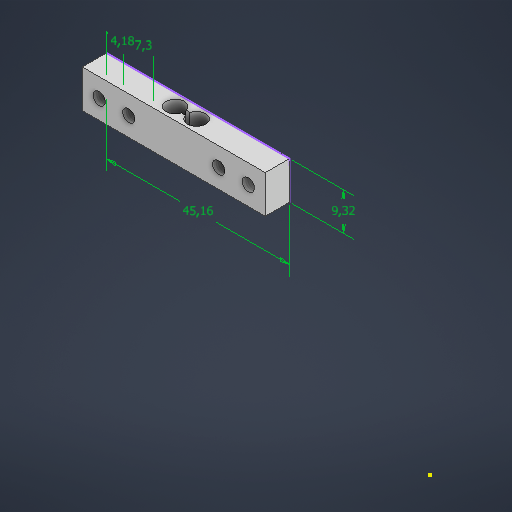
# Autodesk Inventor part: load_cell
Saved by Autodesk Inventor 2026 (Build 300175000, 175)
## iProperties
Created: 2025-04-15
Part Number: load_cell
Material: Generic
Document SubType Name: Modeling
Designer: Paul Juschitz
Density: 1 g/cm^3
Appearance: Default
load_cell_length: 45,160 mm
load_cell_width: 9,320 mm
load_cell_hole_inset: 4,180 mm
load_cell_hole_spacing: 7,300 mm
load_cell_height: 5,990 mm
Author: Paul Juschitz
Autodesk Inventor part; units mm, degrees
ref_plane "YZ Plane" through (0, 0, 0) normal (1, 0, 0) x (0, 1, 0)
ref_plane "XZ Plane" through (0, 0, 0) normal (0, 1, 0) x (-1, 0, 0)
ref_plane "XY Plane" through (0, 0, 0) normal (0, 0, 1) x (1, 0, 0)
sketch "Sketch1" plane through (0, 0, 0) normal (0, 0, 1) x (1, 0, 0)
  line L0 (-79.767, 50.3169) -> (-34.607, 50.3169)
  line L1 (-34.607, 50.3169) -> (-34.607, 40.9969)
  line L2 (-34.607, 40.9969) -> (-79.767, 40.9969)
  line L3 (-79.767, 40.9969) -> (-79.767, 50.3169)
  line L4 (-57.187, 40.9969) -> (-57.187, 50.3169)
  point P0 (0, 0)
  point P1 (-75.587, 45.6569)
  point P2 (-79.767, 45.6569)
  point P3 (-68.287, 45.6569)
  point P4 (-38.787, 45.6569)
  point P5 (-46.087, 45.6569)
  dimension "load_cell_length" = 45.16
  dimension "load_cell_width" = 9.32
  dimension "load_cell_hole_inset" = 4.18
  dimension "load_cell_hole_spacing" = 7.3
  constraints: 10 end point, 3 midpoint, 2 parallel, 2 symmetric about line, 1 horizontal, 1 perpendicular
  measures "load_cell_length" distance of L1.end L2.end
  measures "load_cell_width" distance of L0.end L1.end
  measures "load_cell_hole_inset" distance of point (-79.767, 45.657) point (-75.587, 45.657)
  measures "load_cell_hole_spacing" distance of point (-68.287, 45.657) point (-75.587, 45.657)
extrude "Extrusion1" add sketch "Sketch1" along normal blind 5.99
hole "Hole1" at (-38.787, 45.6569, 0) at (-46.087, 45.6569, 0) at (-68.287, 45.6569, 0) at (-75.587, 45.6569, 0) direction (0, 0, 1) diameter 3 end through all
thread "Thread1" size "M3x0.5" class "6H" standard "ANSI Metric M Profile" full length
thread "Thread2" size "M3x0.5" class "6H" standard "ANSI Metric M Profile" full length
thread "Thread3" size "M3x0.5" class "6H" standard "ANSI Metric M Profile" full length
thread "Thread4" size "M3x0.5" class "6H" standard "ANSI Metric M Profile" full length
sketch "Sketch2" plane through (-79.767, 50.3169, 0) normal (0, 1, 0) x (1, 0, 0)
  line L0 (0, 0) -> (45.16, 0)
  line L1 (45.16, -5.99) -> (0, -5.99)
  arc A0 (23.0312, -3.4698) -> (23.0312, -2.5202) centre (25.2213, -2.995) ccw
  arc A1 (22.1288, -2.5202) -> (22.1288, -3.4698) centre (19.9387, -2.995) ccw
  arc A2 (22.1288, -3.4698) -> (23.0312, -3.4698) centre (22.58, -2.995) ccw
  arc A3 (23.0312, -2.5202) -> (22.1288, -2.5202) centre (22.58, -2.995) ccw
  point P0 (79.767, 0)
  constraints: 8 point on circle, 4 centre point, 4 end point, 1 coincident, 1 horizontal, 1 parallel
extrude "Extrusion2" cut sketch "Sketch2" against normal through all
body "Solid1"
